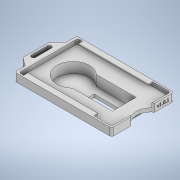
# Autodesk Inventor part: badge
Saved by Autodesk Inventor 2020 (Build 240168000, 168)
## iProperties
Created: 2019-12-22
Part Number: badge
Material: Generic
Document SubType Name: Modeling
Designer: user
Density: 1 g/cm^3
Appearance: Default
Author: user
## iProperties of the stored document _3DPrint.ipt
Created: 2019-12-23
Part Number: _3DPrint
Material: Generic
Document SubType Name: Modeling
Designer: user
Density: 1 g/cm^3
Appearance: Default
Author: user
Autodesk Inventor part; units mm, degrees
ref_plane "YZ Plane" through (0, 0, 0) normal (1, 0, 0) x (0, 1, 0)
ref_plane "XZ Plane" through (0, 0, 0) normal (0, 1, 0) x (-1, 0, 0)
ref_plane "XY Plane" through (0, 0, 0) normal (0, 0, 1) x (1, 0, 0)
sketch "Sketch1" plane through (0, 0, 0) normal (0, 1, 0) x (-1, 0, 0)
  line L0 (11.6176, 24.7873) -> (-76.1824, 24.7873)
  line L1 (-76.1824, -34.0127) -> (11.6176, -34.0127)
  line L2 (13.6176, 14.7873) -> (20.7928, 9.5772)
  line L3 (21.6176, 7.9589) -> (21.6176, -15.1843)
  line L4 (21.0318, -16.5985) -> (13.6176, -24.0127)
  line L5 (15.7066, 2.7873) -> (15.7066, -12.0127)
  line L6 (19.6176, -12.0127) -> (19.6176, 2.7873)
  arc A0 (17.6176, -14.0127) -> (19.6176, -12.0127) centre (17.6176, -12.0127) ccw
  arc A1 (15.7066, -12.0127) -> (17.7066, -14.0127) centre (17.7066, -12.0127) ccw
  arc A2 (17.7066, 4.7873) -> (15.7066, 2.7873) centre (17.7066, 2.7873) ccw
  arc A3 (19.6176, 2.7873) -> (17.6176, 4.7873) centre (17.6176, 2.7873) ccw
  circle A4 centre (-12.3637, -4.6127) radius 18.5
  line L7 (-63.6615, 7.6373) -> (-63.6615, -16.8627)
  line L8 (-61.6615, -18.8627) -> (-24.1615, -18.8627)
  line L9 (-24.1615, 9.6373) -> (-61.6615, 9.6373)
  arc A5 (-63.6615, -16.8627) -> (-61.6615, -18.8627) centre (-61.6615, -16.8627) ccw
  arc A6 (-61.6615, 9.6373) -> (-63.6615, 7.6373) centre (-61.6615, 7.6373) ccw
  line L10 (-28.0615, -0.3627) -> (-53.5615, -0.3627)
  line L11 (-53.5615, -0.3627) -> (-53.5615, -8.8627)
  line L12 (-53.5615, -8.8627) -> (-28.0615, -8.8627)
  line L13 (-28.0615, -8.8627) -> (-28.0615, -0.3627)
  line L14 (-78.1824, 6.7873) -> (-78.1824, 22.7873)
  line L15 (-78.1824, -16.0127) -> (-78.1824, -32.0127)
  line L16 (9.1144, 23.2873) -> (-74.6824, 23.2873)
  line L17 (-74.6824, -32.5127) -> (9.1144, -32.5127)
  line L18 (11.1144, -30.5127) -> (11.1144, 21.2873)
  line L19 (-76.6824, 21.2873) -> (-76.6824, 5.6132)
  line L20 (-76.6824, -30.5127) -> (-76.6824, -14.8386)
  line L21 (13.6176, 22.7873) -> (13.6176, 14.7873)
  line L22 (13.6176, -24.0127) -> (13.6176, -32.0127)
  arc A7 (-78.1824, -32.0127) -> (-76.1824, -34.0127) centre (-76.1824, -32.0127) ccw
  arc A8 (-76.6824, -30.5127) -> (-74.6824, -32.5127) centre (-74.6824, -30.5127) ccw
  arc A9 (-74.6824, 23.2873) -> (-76.6824, 21.2873) centre (-74.6824, 21.2873) ccw
  arc A10 (-76.1824, 24.7873) -> (-78.1824, 22.7873) centre (-76.1824, 22.7873) ccw
  arc A11 (13.6176, 22.7873) -> (11.6176, 24.7873) centre (11.6176, 22.7873) ccw
  arc A12 (11.1144, 21.2873) -> (9.1144, 23.2873) centre (9.1144, 21.2873) ccw
  arc A13 (9.1144, -32.5127) -> (11.1144, -30.5127) centre (9.1144, -30.5127) ccw
  arc A14 (11.6176, -34.0127) -> (13.6176, -32.0127) centre (11.6176, -32.0127) ccw
  arc A15 (21.0318, -16.5985) -> (21.6176, -15.1843) centre (19.6176, -15.1843) ccw
  arc A16 (21.6176, 7.9589) -> (20.7928, 9.5772) centre (19.6176, 7.9589) ccw
  arc A17 (-78.1824, -16.0127) -> (-78.1824, 6.7873) centre (-85.8962, -4.6127) ccw
  point P0 (0, 0)
  point P1 (13.6176, 24.7873)
  point P2 (-78.1824, -34.0127)
  point P3 (-78.1824, 24.7873)
  point P4 (13.6176, -34.0127)
  point P5 (21.6176, -16.0127)
  point P6 (-63.6615, -18.8627)
  point P7 (17.6621, 4.7868)
  point P8 (17.6621, -14.0122)
  dimension "d1" = 91.8
  dimension "d2" = 8
  dimension "d11" = 10
  dimension "d12" = 10
  dimension "d14" = 2
  dimension "d16" = 2
  dimension "d17" = 2
  dimension "d19" = 18
  dimension "d20" = 37
  dimension "d24" = 39.5
  dimension "d25" = 28.5
  dimension "d26" = 2
  dimension "d28" = 10
  dimension "d32" = 10
  dimension "d33" = 10.1
  dimension "d34" = 25.5
  dimension "d36" = 1.5
  dimension "d37" = 1.5
  dimension "d40" = 1.5
  dimension "d41" = 2
  dimension "d84" = 55.8
  dimension "d85" = 10
  dimension "d86" = 10
  dimension "d87" = 27.9
  dimension "d88" = 27.9
  dimension "d89" = 18
  dimension "d104" = 87.7968
  dimension "d105" = 2.5032
  dimension "d106" = 8
  dimension "d107" = 13.65
  dimension "d108" = 13.65
  dimension "d110" = 13.7646
  dimension "d116" = 1.5
  constraints: 46 end point, 38 point on circle, 28 tangent, 18 centre point, 13 point on line, 12 equal radius, 8 equal length, 5 vertical, 3 horizontal, 3 perpendicular, 2 horizontal alignment, 8 other
  measures "d1" distance of point (-78.182, -34.013) point (13.618, -34.013)
  measures "d2" horizontal distance of point (21.618, -16.013) L4.end
  measures "d14" distance between parallel lines of L3 L6
  measures "d16" radius of A0
  measures "d17" radius of A1
  measures "d19" distance of point (-78.182, 24.787) L14.start
  measures "d20" diameter of A4
  measures "d24" distance of point (-63.662, -18.863) L8.end
  measures "d25" distance of L8.end L9.start
  measures "d26" radius of A5
  measures "d28" distance between parallel lines of L8 L12
  measures "d32" distance between parallel lines of L10 L9
  measures "d33" distance between parallel lines of L7 L11
  measures "d34" distance of L11.end L12.end
  measures "d36" distance between parallel lines of L0 L16
  measures "d37" distance between parallel lines of L1 L17
  measures "d40" distance between parallel lines of L15 L20
  measures "d41" radius of A7
  measures "d84" distance between parallel lines of L17 L16
  measures "d85" distance of point (13.618, 24.787) L2.start
  measures "d86" distance of point (13.618, -34.013) L4.end
  measures "d87" distance from line of A4.centre L17
  measures "d88" distance from line of L16 A4.centre
  measures "d89" distance of L15.start point (-78.182, -34.013)
  measures "d104" distance between parallel lines of L19 L18
  measures "d105" distance between parallel lines of L18 L22
  measures "d106" distance between parallel lines of L21 L3
  measures "d107" distance between parallel lines of L16 L9
  measures "d108" distance between parallel lines of L17 L8
  measures "d110" radius of A17
  measures "d116" distance between parallel lines of L19 L14
extrude "OutsideFrame_Ex" add sketch "Sketch1" along normal blind 7.4 contours A11 L21 L2 A16 L3 A15 L4 L22 A14 L1 A7 L15 A17 L20 A8 L17 A13 L18 A12 L16 A9 L19 L14 A10 L0
extrude "CardRidge" add sketch "Sketch1" along normal blind 3.4 contours L19 A9 L16 A12 L18 A13 L17 A8 L20 A17
extrude "TokenBuffer" add sketch "Sketch1" against normal blind 9.6 contours A4 L12 L13 L10 | A4 L10 L11 L12 L8 A5 L7 A6 L9 picked at (-16.6622, -4.6127)
sketch "Sketch4" plane through (0, 0, 0) normal (0, 1, 0) x (1, 0, 0)
  arc A0 (24.1615, 18.8627) -> (24.1615, -9.6373) centre (12.3637, 4.6127) ccw projected
  circle A1 centre (12.3637, 4.6127) radius 15.5
  line L0 (23.0262, -6.6373) -> (60.6615, -6.6373)
  line L1 (60.6615, -6.6373) -> (60.6615, 15.8627)
  line L2 (60.6615, 15.8627) -> (23.0262, 15.8627)
  line L3 (23.0262, 15.8627) -> (23.0262, -6.6373)
  line L4 (61.6615, -9.6373) -> (24.1615, -9.6373) projected
  line L5 (24.1615, 18.8627) -> (61.6615, 18.8627) projected
  line L6 (63.6615, 16.8627) -> (63.6615, -7.6373) projected
  point P0 (0, 0)
  point P1 (23.0262, 15.8627)
  point P2 (23.0262, 15.8627)
  dimension "d56" = 3
  dimension "d57" = 3
  dimension "d58" = 3
  dimension "d59" = 3
  constraints: 8 end point, 2 parallel, 1 coincident, 1 horizontal, 1 perpendicular, 3 other
  measures "d57" distance between parallel lines of L4 L0
  measures "d58" distance between parallel lines of L5 L2
  measures "d59" distance between parallel lines of L6 L1
extrude "TokenCut" cut sketch "Sketch4" against normal blind 6.6
sketch "Sketch5" plane through (74.6824, 7.4, 23.2873) normal (0, 0, -1) x (-1, 0, 0)
  line L0 (-2, 0) -> (0, 0) projected
  line L1 (81.2968, 0) -> (81.2968, -1)
  line L2 (0, 0) -> (83.7968, 0) projected
  line L3 (15, 0) -> (81.2968, 0)
  line L4 (81.2968, 0) -> (81.2968, -1)
  line L5 (81.2968, -1) -> (15, -1)
  line L6 (15, -1) -> (15, 0)
  line L7 (0, -7.4) -> (0, 0) projected
  line L8 (83.7968, -7.4) -> (83.7968, 0) projected
  line L9 (0, -4) -> (83.7968, -4) projected
  point P0 (74.6824, -7.4)
  dimension "d65" = 15
  dimension "d66" = 2.5
  dimension "d67" = 1
  constraints: 10 end point, 2 parallel, 1 horizontal, 1 perpendicular, 1 point on line
  measures "d65" distance between parallel lines of L7 L6
  measures "d66" distance between parallel lines of L8 L1
  measures "d67" distance between parallel lines of L5 L2
extrude "LeftSlider" add sketch "Sketch5" along normal blind 4 contours L1 L5 L6 L2
sketch "Sketch6" plane through (-9.1144, 7.4, -32.5127) normal (0, 0, 1) x (1, 0, 0)
  line L0 (85.2968, 0) -> (-2.5032, 0) projected
  line L1 (2.5, 0) -> (68.7968, 0)
  line L2 (68.7968, 0) -> (68.7968, -1)
  line L3 (68.7968, -1) -> (2.5, -1)
  line L4 (2.5, -1) -> (2.5, 0)
  line L5 (0, -4) -> (0, 0) projected
  line L6 (83.7968, -4) -> (83.7968, 0) projected
  point P0 (9.1144, -7.4)
  point P1 (0, -7.4)
  point P2 (83.7968, -7.4)
  dimension "d71" = 2.5
  dimension "d72" = 15
  dimension "d73" = 1
  constraints: 8 end point, 2 parallel, 1 horizontal, 1 perpendicular, 1 point on line
  measures "d71" distance between parallel lines of L5 L4
  measures "d72" distance between parallel lines of L6 L2
  measures "d73" distance between parallel lines of L3 L0
extrude "RightSlider" add sketch "Sketch6" along normal blind 4
sketch "Sketch12" plane through (0, 0, 0) normal (0, 1, 0) x (1, 0, 0)
  arc A0 (23.0262, 15.8627) -> (23.0262, -6.6373) centre (12.3637, 4.6127) ccw projected
  circle A1 centre (12.3637, 4.6127) radius 15.5
  circle A2 centre (12.3637, 4.6127) radius 18.5
  line L0 (61.6615, -9.6373) -> (24.1615, -9.6373) projected
  line L1 (24.1615, -9.6373) -> (61.6615, -9.6373)
  line L2 (63.6615, 16.8627) -> (63.6615, -7.6373) projected
  arc A3 (61.6615, -9.6373) -> (63.6615, -7.6373) centre (61.6615, -7.6373) ccw
  line L3 (60.6615, -6.6373) -> (23.0262, -6.6373) projected
  line L4 (23.0262, -6.6373) -> (60.6615, -6.6373)
  line L5 (60.6615, 15.8627) -> (60.6615, -6.6373) projected
  line L6 (60.6615, -6.6373) -> (60.6615, 15.8627)
  line L7 (23.0262, 15.8627) -> (60.6615, 15.8627) projected
  line L8 (60.6615, 15.8627) -> (23.0262, 15.8627)
  line L9 (63.6615, -7.6373) -> (64.1048, 16.8627)
  line L10 (63.6615, 16.8627) -> (63.6615, -7.6373) projected
  line L11 (63.6615, -7.6373) -> (63.6615, 16.8627)
  line L12 (24.1615, 18.8627) -> (61.6615, 18.8627) projected
  arc A4 (63.6615, 16.8627) -> (61.6615, 18.8627) centre (61.6615, 16.8627) ccw
  line L13 (61.6615, 18.8627) -> (24.1615, 18.8627)
  point P0 (0, 0)
  point P1 (27.05, 15.8627)
  point P2 (27.05, -6.6373)
  constraints: 14 end point, 4 centre point, 4 point on circle, 2 coincident, 2 horizontal, 2 perpendicular, 1 collinear, 1 tangent
extrude "Extrusion13" add sketch "Sketch12" along normal blind 3.4 contours A2 L12 A4 L2 A3 L0 L3 L5 L7
extrude "Extrusion14" add sketch "Sketch12" along normal blind 3.4 contours A0 L3 A2 L7
sketch "Sketch15" plane through (78.1824, 0, -16.0127) normal (1, 0, 0) x (0, 0, -1)
  line L0 (2.191, 5.3205) -> (13.1828, 5.3205) construction
  line L1 (13.1828, 5.3205) -> (13.1828, 0.2382) construction
  line L2 (13.1828, 0.2382) -> (2.191, 0.2382) construction
  line L3 (2.191, 0.2382) -> (2.191, 5.3205) construction
  line L4 (4.2658, 4.498) -> (3.4038, 2.2107)
  line L5 (3.4038, 2.2107) -> (3.058, 2.2107)
  line L6 (3.058, 2.2107) -> (2.2033, 4.498)
  line L7 (2.2033, 4.498) -> (2.6208, 4.498)
  line L8 (2.6208, 4.498) -> (3.2457, 2.7368)
  line L9 (3.2457, 2.7368) -> (3.8657, 4.498)
  line L10 (3.8657, 4.498) -> (4.2658, 4.498)
  line L11 (6.227, 2.2107) -> (4.74, 2.2107)
  line L12 (4.74, 2.2107) -> (4.74, 2.522)
  line L13 (4.74, 2.522) -> (5.2933, 2.522)
  line L14 (5.2933, 2.522) -> (5.2933, 4.5647)
  line L15 (5.2933, 4.5647) -> (4.74, 4.5647)
  line L16 (4.74, 4.5647) -> (4.74, 4.8438)
  spline S0 degree 2 poles (4.74, 4.8438) (5.0537, 4.8438) (5.3501, 5.0216) (5.3699, 5.2686) knots 0 0 0 1 2 2 2
  line L17 (5.3699, 5.2686) -> (5.6861, 5.2686)
  line L18 (5.6861, 5.2686) -> (5.6861, 2.522)
  line L19 (5.6861, 2.522) -> (6.227, 2.522)
  line L20 (6.227, 2.522) -> (6.227, 2.2107)
  line L21 (7.4422, 2.2107) -> (6.9532, 2.2107)
  line L22 (6.9532, 2.2107) -> (6.9532, 2.7937)
  line L23 (6.9532, 2.7937) -> (7.4422, 2.7937)
  line L24 (7.4422, 2.7937) -> (7.4422, 2.2107)
  spline S1 degree 2 poles (9.9542, 3.7347) (9.9542, 2.9147) (9.4775, 2.1465) (8.9811, 2.1465) knots 0 0 0 1 2 2 2
  spline S2 degree 2 poles (8.9811, 2.1465) (8.4772, 2.1465) (8.0054, 2.9295) (8.0054, 3.7323) knots 0 0 0 1 2 2 2
  spline S3 degree 2 poles (8.0054, 3.7323) (8.0054, 4.5573) (8.4821, 5.3205) (8.9811, 5.3205) knots 0 0 0 1 2 2 2
  spline S4 degree 2 poles (8.9811, 5.3205) (9.4825, 5.3205) (9.9542, 4.5301) (9.9542, 3.7347) knots 0 0 0 1 2 2 2
  spline S5 degree 2 poles (9.4306, 2.806) (9.4899, 2.9567) (9.5393, 3.421) (9.5393, 3.7347) knots 0 0 0 1 2 2 2
  spline S6 degree 2 poles (9.5393, 3.7347) (9.5393, 4.0484) (9.4899, 4.5103) (9.4281, 4.6659) knots 0 0 0 1 2 2 2
  spline S7 degree 2 poles (9.4281, 4.6659) (9.3664, 4.8215) (9.1515, 4.9821) (8.9811, 4.9821) knots 0 0 0 1 2 2 2
  spline S8 degree 2 poles (8.9811, 4.9821) (8.8106, 4.9821) (8.5908, 4.8215) (8.5266, 4.661) knots 0 0 0 1 2 2 2
  spline S9 degree 2 poles (8.5266, 4.661) (8.4648, 4.5054) (8.4204, 4.0311) (8.4204, 3.7323) knots 0 0 0 1 2 2 2
  spline S10 degree 2 poles (8.4204, 3.7323) (8.4204, 3.4112) (8.4599, 2.9814) (8.5241, 2.8134) knots 0 0 0 1 2 2 2
  spline S11 degree 2 poles (8.5241, 2.8134) (8.5834, 2.6553) (8.8032, 2.4849) (8.9811, 2.4849) knots 0 0 0 1 2 2 2
  spline S12 degree 2 poles (8.9811, 2.4849) (9.149, 2.4849) (9.3689, 2.6455) (9.4306, 2.806) knots 0 0 0 1 2 2 2
  line L25 (10.9991, 2.2107) -> (10.51, 2.2107)
  line L26 (10.51, 2.2107) -> (10.51, 2.7937)
  line L27 (10.51, 2.7937) -> (10.9991, 2.7937)
  line L28 (10.9991, 2.7937) -> (10.9991, 2.2107)
  line L29 (13.3406, 2.2107) -> (11.8537, 2.2107)
  line L30 (11.8537, 2.2107) -> (11.8537, 2.522)
  line L31 (11.8537, 2.522) -> (12.407, 2.522)
  line L32 (12.407, 2.522) -> (12.407, 4.5647)
  line L33 (12.407, 4.5647) -> (11.8537, 4.5647)
  line L34 (11.8537, 4.5647) -> (11.8537, 4.8438)
  spline S13 degree 2 poles (11.8537, 4.8438) (12.1674, 4.8438) (12.4638, 5.0216) (12.4835, 5.2686) knots 0 0 0 1 2 2 2
  line L35 (12.4835, 5.2686) -> (12.7997, 5.2686)
  line L36 (12.7997, 5.2686) -> (12.7997, 2.522)
  line L37 (12.7997, 2.522) -> (13.3406, 2.522)
  line L38 (13.3406, 2.522) -> (13.3406, 2.2107)
  point P0 (-16.0127, 0)
  constraints: 2 other
emboss "Emboss2" sketch "Sketch15" operation cut depth 1 direction (-1, 0, 0)
equation "\"d12\" = d11"
equation "\"d86\" = d85"
equation "\"d87\" = d88"
equation "\"d89\" = d19"
body "Solid3"
